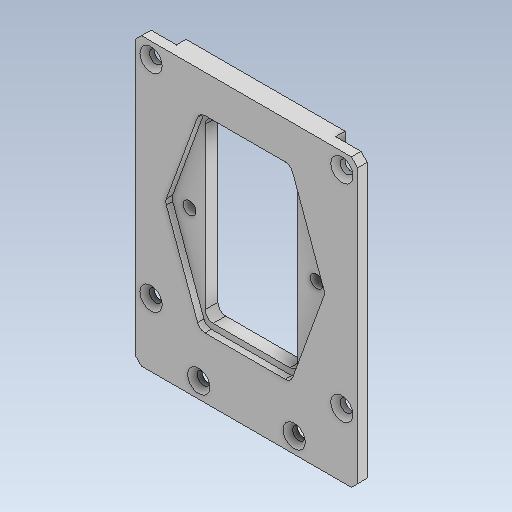
# Autodesk Inventor part: 10-06-015 Suport conector cablu
Saved by Autodesk Inventor 2020 (Build 240168000, 168)
## iProperties
Created: 2020-01-17
Part Number: 10-06-015 Suport conector cablu
Material: Generic
Document SubType Name: Modeling
Designer: iuliu
Density: 1 g/cm^3
Appearance: Default
Description: Capac priza
Mass: 18.5853 g
Surface Area: 121.574 cm^2
Volume: 18.5853 cm^3
Author: iuliu
Subject: 050
Autodesk Inventor part; units mm, degrees
ref_plane "YZ Plane" through (0, 0, 0) normal (1, 0, 0) x (0, 1, 0)
ref_plane "XZ Plane" through (0, 0, 0) normal (0, 1, 0) x (-1, 0, 0)
ref_plane "XY Plane" through (0, 0, 0) normal (0, 0, 1) x (1, 0, 0)
sketch "Sketch1" plane through (0, 0, 0) normal (0, 0, 1) x (1, 0, 0)
  line L0 (-35, 45) -> (35, 45)
  line L1 (35, 45) -> (35, -45)
  line L2 (35, -45) -> (-35, -45)
  line L3 (-35, -45) -> (-35, 45)
  point P0 (0, 0)
  point P1 (0, 45)
  point P2 (-35, 0)
  dimension "d0" = 70
  dimension "d1" = 90
  constraints: 8 end point, 2 midpoint, 2 parallel, 1 horizontal, 1 horizontal alignment, 1 perpendicular, 1 vertical alignment
  measures "d0" distance of L0.start L0.end
  measures "d1" distance of L2.end L0.start
extrude "Extrusion1" add sketch "Sketch1" along normal blind 23
sketch "Sketch2" plane through (0, 0, 23) normal (0, 0, 1) x (1, 0, 0)
  circle A0 centre (-20.425, 3.625) radius 3.15
  circle A1 centre (19.575, 3.625) radius 3.15
  line L0 (12.1727, -25.475) -> (-13.0227, -25.475)
  arc A2 (-14.903, -24.1567) -> (-13.0227, -25.475) centre (-13.0227, -23.475) ccw
  line L1 (-14.903, -24.1567) -> (-24.7279, 2.9433)
  arc A3 (-24.7279, 4.3067) -> (-24.7279, 2.9433) centre (-22.8476, 3.625) ccw
  line L2 (-24.7279, 4.3067) -> (-14.903, 31.4067)
  arc A4 (-13.0227, 32.725) -> (-14.903, 31.4067) centre (-13.0227, 30.725) ccw
  line L3 (-13.0227, 32.725) -> (12.1727, 32.725)
  arc A5 (14.053, 31.4067) -> (12.1727, 32.725) centre (12.1727, 30.725) ccw
  line L4 (14.053, 31.4067) -> (23.8779, 4.3067)
  arc A6 (23.8779, 2.9433) -> (23.8779, 4.3067) centre (21.9976, 3.625) ccw
  line L5 (23.8779, 2.9433) -> (14.053, -24.1567)
  arc A7 (12.1727, -25.475) -> (14.053, -24.1567) centre (12.1727, -23.475) ccw
  line L6 (-12.5, 30.85) -> (11.65, 30.85)
  arc A8 (13.65, 28.85) -> (11.65, 30.85) centre (11.65, 28.85) ccw
  line L7 (13.65, 28.85) -> (13.65, -21.6)
  arc A9 (11.65, -23.6) -> (13.65, -21.6) centre (11.65, -21.6) ccw
  line L8 (11.65, -23.6) -> (-12.5, -23.6)
  arc A10 (-14.5, -21.6) -> (-12.5, -23.6) centre (-12.5, -21.6) ccw
  line L9 (-14.5, -21.6) -> (-14.5, 28.85)
  arc A11 (-12.5, 30.85) -> (-14.5, 28.85) centre (-12.5, 28.85) ccw
  line L10 (11.875, -14) -> (11.875, -4.28)
  arc A12 (11.875, -4.28) -> (9.875, -2.28) centre (9.875, -4.28) ccw
  line L11 (9.875, -2.28) -> (-10.725, -2.28)
  arc A13 (-10.725, -2.28) -> (-12.725, -4.28) centre (-10.725, -4.28) ccw
  line L12 (-12.725, -4.28) -> (-12.725, -14)
  line L13 (-12.725, -14) -> (-7.725, -19)
  line L14 (-7.725, -19) -> (6.875, -19)
  line L15 (6.875, -19) -> (11.875, -14)
  line L16 (0.575, -12.25) -> (0.575, -15.75)
  line L17 (0.575, -15.75) -> (-1.425, -15.75)
  line L18 (-1.425, -15.75) -> (-1.425, -12.25)
  line L19 (-1.425, -12.25) -> (0.575, -12.25)
  line L20 (-6.3111, -5.53) -> (-6.3111, -9.03)
  line L21 (-6.3111, -9.03) -> (-8.3111, -9.03)
  line L22 (-8.3111, -9.03) -> (-8.3111, -5.53)
  line L23 (-8.3111, -5.53) -> (-6.3111, -5.53)
  line L24 (5.4611, -9.03) -> (5.4611, -5.53)
  line L25 (5.4611, -5.53) -> (7.4611, -5.53)
  line L26 (7.4611, -5.53) -> (7.4611, -9.03)
  line L27 (7.4611, -9.03) -> (5.4611, -9.03)
  line L28 (11.65, 31.35) -> (-12.5, 31.35)
  arc A14 (-12.5, 31.35) -> (-15, 28.85) centre (-12.5, 28.85) ccw
  line L29 (-15, 28.85) -> (-15, -21.6)
  arc A15 (-15, -21.6) -> (-12.5, -24.1) centre (-12.5, -21.6) ccw
  line L30 (-12.5, -24.1) -> (11.65, -24.1)
  arc A16 (11.65, -24.1) -> (14.15, -21.6) centre (11.65, -21.6) ccw
  line L31 (14.15, -21.6) -> (14.15, 28.85)
  arc A17 (14.15, 28.85) -> (11.65, 31.35) centre (11.65, 28.85) ccw
  dimension "d90" = 0.5
  constraints: 64 end point, 32 point on circle, 18 centre point, 12 horizontal, 10 vertical, 81 other
  measures "d90" distance between parallel lines of L6 L28
extrude "Extrusion2" cut sketch "Sketch2" against normal through all contours L6 A8 L7 A9 L8 A10 L9 A11 | L15 L14 L13 L12 A13 L11 A12 L10 | L16 L17 L18 L19 | L20 L21 L22 L23 | L24 L25 L26 L27 | A17 L31 A16 L30 A15 L29 A14 L28
sketch "Sketch3" plane through (0, 0, 23) normal (0, 0, 1) x (1, 0, 0)
  circle A0 centre (-20.425, 3.625) radius 3.15
  circle A1 centre (19.575, 3.625) radius 3.15
  line L0 (12.1727, -25.475) -> (-13.0227, -25.475)
  arc A2 (-14.903, -24.1567) -> (-13.0227, -25.475) centre (-13.0227, -23.475) ccw
  line L1 (-14.903, -24.1567) -> (-24.7279, 2.9433)
  arc A3 (-24.7279, 4.3067) -> (-24.7279, 2.9433) centre (-22.8476, 3.625) ccw
  line L2 (-24.7279, 4.3067) -> (-14.903, 31.4067)
  arc A4 (-13.0227, 32.725) -> (-14.903, 31.4067) centre (-13.0227, 30.725) ccw
  line L3 (-13.0227, 32.725) -> (12.1727, 32.725)
  arc A5 (14.053, 31.4067) -> (12.1727, 32.725) centre (12.1727, 30.725) ccw
  line L4 (14.053, 31.4067) -> (23.8779, 4.3067)
  arc A6 (23.8779, 2.9433) -> (23.8779, 4.3067) centre (21.9976, 3.625) ccw
  line L5 (23.8779, 2.9433) -> (14.053, -24.1567)
  arc A7 (12.1727, -25.475) -> (14.053, -24.1567) centre (12.1727, -23.475) ccw
  line L6 (-12.5, 30.85) -> (11.65, 30.85)
  arc A8 (13.65, 28.85) -> (11.65, 30.85) centre (11.65, 28.85) ccw
  line L7 (13.65, 28.85) -> (13.65, -21.6)
  arc A9 (11.65, -23.6) -> (13.65, -21.6) centre (11.65, -21.6) ccw
  line L8 (11.65, -23.6) -> (-12.5, -23.6)
  arc A10 (-14.5, -21.6) -> (-12.5, -23.6) centre (-12.5, -21.6) ccw
  line L9 (-14.5, -21.6) -> (-14.5, 28.85)
  arc A11 (-12.5, 30.85) -> (-14.5, 28.85) centre (-12.5, 28.85) ccw
  line L10 (11.875, -14) -> (11.875, -4.28)
  arc A12 (11.875, -4.28) -> (9.875, -2.28) centre (9.875, -4.28) ccw
  line L11 (9.875, -2.28) -> (-10.725, -2.28)
  arc A13 (-10.725, -2.28) -> (-12.725, -4.28) centre (-10.725, -4.28) ccw
  line L12 (-12.725, -4.28) -> (-12.725, -14)
  line L13 (-12.725, -14) -> (-7.725, -19)
  line L14 (-7.725, -19) -> (6.875, -19)
  line L15 (6.875, -19) -> (11.875, -14)
  line L16 (0.575, -12.25) -> (0.575, -15.75)
  line L17 (0.575, -15.75) -> (-1.425, -15.75)
  line L18 (-1.425, -15.75) -> (-1.425, -12.25)
  line L19 (-1.425, -12.25) -> (0.575, -12.25)
  line L20 (-6.3111, -5.53) -> (-6.3111, -9.03)
  line L21 (-6.3111, -9.03) -> (-8.3111, -9.03)
  line L22 (-8.3111, -9.03) -> (-8.3111, -5.53)
  line L23 (-8.3111, -5.53) -> (-6.3111, -5.53)
  line L24 (5.4611, -9.03) -> (5.4611, -5.53)
  line L25 (5.4611, -5.53) -> (7.4611, -5.53)
  line L26 (7.4611, -5.53) -> (7.4611, -9.03)
  line L27 (7.4611, -9.03) -> (5.4611, -9.03)
  line L28 (12.1727, 33.225) -> (-13.0227, 33.225)
  arc A14 (-13.0227, 33.225) -> (-15.373, 31.5771) centre (-13.0227, 30.725) ccw
  line L29 (-15.373, 31.5771) -> (-25.1979, 4.4771)
  arc A15 (-25.1979, 4.4771) -> (-25.1979, 2.7729) centre (-22.8476, 3.625) ccw
  line L30 (-25.1979, 2.7729) -> (-15.373, -24.3271)
  arc A16 (-15.373, -24.3271) -> (-13.0227, -25.975) centre (-13.0227, -23.475) ccw
  line L31 (-13.0227, -25.975) -> (12.1727, -25.975)
  arc A17 (12.1727, -25.975) -> (14.523, -24.3271) centre (12.1727, -23.475) ccw
  line L32 (14.523, -24.3271) -> (24.3479, 2.7729)
  arc A18 (24.3479, 2.7729) -> (24.3479, 4.4771) centre (21.9976, 3.625) ccw
  line L33 (24.3479, 4.4771) -> (14.523, 31.5771)
  arc A19 (14.523, 31.5771) -> (12.1727, 33.225) centre (12.1727, 30.725) ccw
  dimension "d91" = 0.5
  constraints: 68 end point, 36 point on circle, 20 centre point, 12 horizontal, 10 vertical, 85 other
  measures "d91" distance between parallel lines of L3 L28
extrude "Extrusion3" cut sketch "Sketch3" against normal blind 2 contours A0 | A1 | L0 A2 L1 A3 L2 A4 L3 A5 L4 A6 L5 A7 | L6 A8 L7 A9 L8 A10 L9 A11 | L15 L14 L13 L12 A13 L11 A12 L10 | L16 L17 L18 L19 | L20 L21 L22 L23 | L24 L25 L26 L27 | A19 L33 A18 L32 A17 L31 A16 L30 A15 L29 A14 L28
sketch "Sketch4" plane through (0, 0, 0) normal (0, 0, -1) x (-1, 0, 0)
  line L0 (-25, 45) -> (25, 45)
  line L1 (25, 45) -> (25, -30)
  line L2 (25, -30) -> (-25, -30)
  line L3 (-25, -30) -> (-25, 45)
  line L4 (-35, -45) -> (-35, 45) projected
  line L5 (35, -45) -> (-35, -45) projected
  line L6 (-35, 45) -> (35, 45) projected
  line L7 (35, 45) -> (35, -45) projected
  point P0 (0, 0)
  point P1 (45, -30)
  point P2 (-25, 45)
  point P3 (0, -30)
  point P4 (0, -45)
  point P5 (25, 45)
  dimension "d11" = 15
  dimension "d89" = 10
  constraints: 8 end point, 2 midpoint, 2 parallel, 1 collinear, 1 horizontal, 1 perpendicular, 1 vertical alignment
  measures "d11" distance between parallel lines of L5 L2
  measures "d89" distance between parallel lines of L4 L3
extrude "Extrusion4" cut sketch "Sketch4" against normal blind 20 contours L3 L2 L1 L6 L7 L5 L4
sketch "Sketch6" plane through (0, 0, 23) normal (0, 0, 1) x (1, 0, 0)
  circle A0 centre (-19.865, 3.655) radius 1.6 projected
  circle A1 centre (20.135, 3.655) radius 1.6 projected
  point P0 (0, 0)
hole "Hole1" at (20.135, 3.655, 23) at (-19.865, 3.655, 23) direction (0, 0, -1) diameter 4 end through all
sketch "Sketch5" plane through (0, 0, 0) normal (0, 0, -1) x (-1, 0, 0)
  line L0 (-20, 45) -> (45, 45)
  line L1 (-20, 0) -> (-20, 45)
  line L2 (-25, 45) -> (35, 45) projected
  line L3 (-25, 45) -> (-25, -30) projected
  line L4 (-25, -30) -> (25, -30) projected
  line L5 (14.9072, -25) -> (34.9072, -25)
  line L6 (35, -30) -> (14.9072, -30)
  line L7 (14.9072, -25) -> (14.9072, -30)
  line L8 (-25, 0) -> (-20, 0)
  line L9 (35, 45) -> (35, -30)
  point P0 (-20, -30)
  point P1 (14.9072, -30)
  point P2 (-20, 45)
  point P3 (14.9072, -30)
  point P4 (35, 45)
  dimension "d17" = 5
  dimension "d35" = 5
  dimension "d80" = 30
  dimension "d96" = 20.0928
  constraints: 14 end point, 2 collinear, 2 horizontal, 2 perpendicular, 2 point on line, 1 parallel, 1 vertical
  measures "d17" distance between parallel lines of L3 L1
  measures "d35" distance of L5.start L6.end
  measures "d80" distance between parallel lines of L4 L8
  measures "d96" distance of L6.start L6.end
extrude "Extrusion5" cut sketch "Sketch5" against normal blind 17
sketch "Sketch9" plane through (0, 0, 17) normal (0, 0, -1) x (-1, 0, 0)
  line L0 (-25, 45) -> (25, 45) projected
  line L1 (25, -30) -> (-25, -30) projected
  line L2 (-9.15, -24.1) -> (20, -24.1)
  line L3 (20, -24.1) -> (20, -30)
  line L4 (20, -30) -> (-9.15, -30)
  line L5 (-9.15, -30) -> (-9.15, -24.1)
  line L6 (-25, -30) -> (-25, 45) projected
  line L7 (25, 45) -> (25, -30) projected
  line L8 (-14.15, 28.85) -> (-14.15, -21.6) projected
  arc A0 (-11.65, 31.35) -> (-14.15, 28.85) centre (-11.65, 28.85) ccw projected
  line L9 (12.5, 31.35) -> (-11.65, 31.35) projected
  arc A1 (15, 28.85) -> (12.5, 31.35) centre (12.5, 28.85) ccw projected
  line L10 (15, -21.6) -> (15, 28.85) projected
  arc A2 (12.5, -24.1) -> (15, -21.6) centre (12.5, -21.6) ccw projected
  line L11 (-11.65, -24.1) -> (12.5, -24.1) projected
  arc A3 (-14.15, -21.6) -> (-11.65, -24.1) centre (-11.65, -21.6) ccw projected
  point P0 (0, 0)
  point P1 (-9.15, -30)
  point P2 (20, -30)
  constraints: 8 end point, 2 parallel, 1 collinear, 1 horizontal, 1 perpendicular
extrude "Extrusion6" [suppressed]
sketch "Sketch10" plane through (-17.5, -24.1, 21) normal (0, 1, 0) x (1, 0, 0)
  line L0 (22.5, 19) -> (2.5, 19)
  line L1 (2.5, 19) -> (2.5, 29)
  line L2 (2.5, 29) -> (22.5, 29)
  line L3 (22.5, 29) -> (22.5, 19)
  point P0 (17.5, 21)
  point P1 (12.5, 29)
  point P2 (12.5, 34)
  dimension "d94" = 10
  constraints: 8 end point, 2 parallel, 1 horizontal, 1 midpoint, 1 perpendicular, 1 vertical alignment
  measures "d94" distance of L0.end L1.end
extrude "Extrusion7" [suppressed]
fillet "Fillet1" [suppressed]
sketch "Sketch11" plane through (0, 0, 23) normal (0, 0, 1) x (1, 0, 0)
  line L0 (-35, -45) -> (35, -45) projected
  line L1 (-35, 45) -> (-35, -45) projected
  line L2 (35, -45) -> (35, 45) projected
  line L3 (35, 45) -> (-35, 45) projected
  point P0 (0, 0)
  point P1 (-15, -40)
  point P2 (15, -40)
  point P3 (30, -25)
  point P4 (30, 40)
  point P5 (-30, 40)
  point P6 (-30, -25)
  dimension "d65" = 5
  dimension "d66" = 20
  dimension "d67" = 20
  dimension "d68" = 5
  dimension "d69" = 5
  dimension "d70" = 20
  dimension "d71" = 5
  dimension "d72" = 5
  dimension "d97" = 5
  constraints: 2 horizontal alignment, 1 vertical alignment
  measures "d65" distance from line of L0 point (-15, -40)
  measures "d66" distance from line of L1 point (-15, -40)
  measures "d67" distance from line of L2 point (15, -40)
  measures "d68" distance from line of L0 point (15, -40)
  measures "d69" distance from line of L2 point (30, -25)
  measures "d70" distance from line of L0 point (30, -25)
  measures "d71" distance from line of L2 point (30, 40)
  measures "d72" distance from line of point (30, 40) L3
  measures "d97" distance from line of L1 point (-30, 40)
hole "Hole4" at (-15, -40, 23) at (15, -40, 23) at (30, -25, 23) at (30, 40, 23) at (-30, 40, 23) at (-30, -25, 23) direction (0, 0, -1) diameter 4 end through all countersink diameter 7 countersink angle 90
chamfer "Chamfer2" distance 2 angle 45 4 edges at (-35, 45, 21.5) (35, 45, 21.5) (35, -45, 21.5) (-35, -45, 21.5)
equation "\"d66\" = d67"
equation "\"d68\" = d65"
equation "\"d69\" = d65"
equation "\"d70\" = d67"
equation "\"d71\" = d65"
equation "\"d97\" = d72"
body "Solid1"
